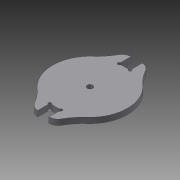
# Autodesk Inventor part: Forward Endcap Outer
Saved by Autodesk Inventor 2016 (Build 200138000, 138)
## iProperties
Created: 2015-06-17
Part Number: Forward Endcap Outer
Material: Generic
Document SubType Name: Modeling
Designer: JR
Density: 1 g/cm^3
Appearance: Default
BattECOD: 40.000 mm
GripLength: 1.500 mm
Author: JR
Autodesk Inventor part; units mm, degrees
ref_plane "YZ Plane" through (0, 0, 0) normal (1, 0, 0) x (0, 1, 0)
ref_plane "XZ Plane" through (0, 0, 0) normal (0, 1, 0) x (-1, 0, 0)
ref_plane "XY Plane" through (0, 0, 0) normal (0, 0, 1) x (1, 0, 0)
sketch "Sketch1" plane through (0, 0, 0) normal (0, 0, 1) x (1, 0, 0)
  circle A0 centre (0, 0) radius 1.5
  circle A1 centre (0, 0) radius 15.875 construction
  line L0 (0, 20) -> (0, -20) construction
  line L1 (-20, 0) -> (20, 0) construction
  line L2 (-2.25, 18.5) -> (0, 18.5)
  line L3 (-6, 25) -> (-3, 25)
  line L4 (-3, 25) -> (-3, 19.25)
  line L5 (2.25, 18.5) -> (0, 18.5)
  line L6 (6, 25) -> (3, 25)
  line L7 (3, 25) -> (3, 19.25)
  line L8 (-2.25, -18.5) -> (0, -18.5)
  line L9 (-6, -25) -> (-3, -25)
  line L10 (-3, -25) -> (-3, -19.25)
  line L11 (2.25, -18.5) -> (0, -18.5)
  line L12 (3, -25) -> (3, -19.25)
  line L13 (6, -25) -> (3, -25)
  arc A2 (-13.3625, 14.881) -> (-13.3625, -14.881) centre (0, 0) ccw
  arc A3 (13.3625, -14.881) -> (13.3625, 14.881) centre (0, 0) ccw
  circle A4 centre (0, 0) radius 20 construction
  arc A5 (-3, 19.25) -> (-2.25, 18.5) centre (-3, 18.5) ccw
  arc A6 (2.25, 18.5) -> (3, 19.25) centre (3, 18.5) ccw
  arc A7 (-2.25, -18.5) -> (-3, -19.25) centre (-3, -18.5) ccw
  arc A8 (3, -19.25) -> (2.25, -18.5) centre (3, -18.5) ccw
  arc A9 (-13.3625, 14.881) -> (-6, 25) centre (-33.4062, 37.2025) ccw
  arc A10 (6, 25) -> (13.3625, 14.881) centre (33.4062, 37.2025) ccw
  arc A11 (-6, -25) -> (-13.3625, -14.881) centre (-33.4062, -37.2025) ccw
  arc A12 (13.3625, -14.881) -> (6, -25) centre (33.4062, -37.2025) ccw
  dimension "d9" = 40
  dimension "d0" = 3
  dimension "d1" = 31.75
  dimension "GripLength" = 1.5
  dimension "d4" = 5
  dimension "d5" = 3
  dimension "d6" = 3
  dimension "d8" = 20
  dimension "d10" = 0.75
  dimension "d15" = 30
  constraints: 28 end point, 22 point on circle, 20 symmetric about line, 12 centre point, 4 coincident, 4 midpoint, 2 horizontal, 2 perpendicular, 2 vertical alignment, 1 horizontal alignment, 1 point on line, 1 tangent, 1 vertical, 8 other
  measures "d0" diameter of A0
  measures "d1" diameter of A1
  measures "GripLength" distance from line of L0.start L2
  measures "d4" distance from line of L3 L0.start
  measures "d5" distance between parallel lines of L0 L4
  measures "d6" distance of L3.start L3.end
  measures "d8" radius of A2
  measures "d10" radius of A5
  measures "d15" radius of A9
extrude "Extrusion1" add sketch "Sketch1" along normal blind 3
fillet "Fillet1" radius 1 8 edges at (-3, 19.25, 1.5) (-2.25, 18.5, 1.5) (2.25, 18.5, 1.5) (3, 19.25, 1.5) (-3, -19.25, 1.5) (-2.25, -18.5, 1.5) (2.25, -18.5, 1.5) (3, -19.25, 1.5)
fillet "Fillet2" radius 5 8 edges at (-13.3625, -14.881, 1.5) (-6, -25, 1.5) (6, -25, 1.5) (13.3625, -14.881, 1.5) (13.3625, 14.881, 1.5) (6, 25, 1.5) (-6, 25, 1.5) (-13.3625, 14.881, 1.5)
equation "\"d1\" = BattOD"
equation "\"BattOD\" = 31.75"
body "Solid1"
